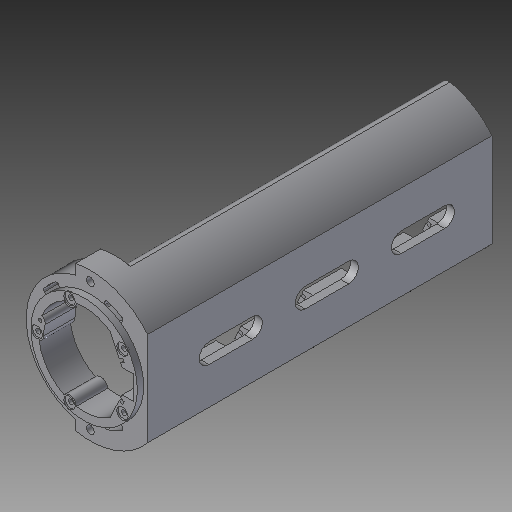
# Autodesk Inventor part: 3212_Bed Rail Base Junction_V1
Saved by Autodesk Inventor 2020 (Build 240168000, 168)
## iProperties
Created: 2019-06-18
Part Number: 3212_Bed Rail Base Junction_V1
Material: Acetal Resin, White
Document SubType Name: Sheet Metal
Designer: MPI
Density: 1.425 g/cm^3
Sheet Metal Rule: Default_mm
Appearance: Smooth - White
Mass: 1109.81 g
Surface Area: 2041.44 cm^2
Volume: 778.816 cm^3
Author: MPI
Autodesk Inventor part; units mm, degrees
ref_plane "YZ Plane" through (0, 0, 0) normal (1, 0, 0) x (0, 1, 0)
ref_plane "XZ Plane" through (0, 0, 0) normal (0, 1, 0) x (-1, 0, 0)
sketch "Sketch1" plane through (0, 0, 0) normal (0, 0, 1) x (1, 0, 0)
  circle A0 centre (0, 0) radius 54
  line L0 (48, 0) -> (-65, 0) construction
  line L1 (0, -54) -> (0, 65) construction
  dimension "d0" = 108
  constraints: 4 end point, 1 coincident, 1 horizontal, 1 perpendicular, 1 vertical alignment, 2 other
extrude "Extrusion1" add sketch "Sketch1" along normal blind 6.35
sketch "Sketch4" plane through (0, 0, 0) normal (0, 0, -1) x (-1, 0, 0)
  line L0 (15, 73.484692) -> (15, 63.245553)
  line L1 (15, -63.245553) -> (15, -73.484692)
  line L2 (-58, 47.549974) -> (-58, -47.549974)
  arc A0 (15, -63.245553) -> (15, 63.245553) centre (0, 0) ccw
  arc A1 (15, 73.484692) -> (-58, 47.549974) centre (0, 0) ccw
  arc A2 (-58, -47.549974) -> (15, -73.484692) centre (0, 0) ccw
  line L3 (-59, 0) -> (82, 0) construction
  line L4 (0, 75) -> (0, -119) construction
  line L5 (-30.377899, -43.384136) -> (-32.673725, -46.662915)
  line L6 (-13.707639, -51.157606) -> (-14.743601, -55.02387)
  line L7 (30.377899, -43.384136) -> (32.673725, -46.662915)
  line L8 (43.384136, -30.377899) -> (46.662915, -32.673725)
  line L9 (43.384136, 30.377899) -> (46.662915, 32.673725)
  line L10 (30.377899, 43.384136) -> (32.673725, 46.662915)
  line L11 (-13.707639, 51.157606) -> (-14.743601, 55.02387)
  line L12 (-30.377899, 43.384136) -> (-32.673725, 46.662915)
  arc A3 (35.51596, -47.112807) -> (47.112807, -35.51596) centre (0, 0) ccw
  arc A4 (30.808045, -40.643135) -> (40.643135, -30.808045) centre (0, 0) ccw
  arc A5 (-32.124383, -49.487615) -> (-17.260557, -56.418731) centre (0, 0) ccw
  arc A6 (-27.655082, -42.850863) -> (-15.049321, -48.729026) centre (0, 0) ccw
  arc A7 (47.112807, 35.51596) -> (35.51596, 47.112807) centre (0, 0) ccw
  arc A8 (-17.260557, 56.418731) -> (-32.124383, 49.487615) centre (0, 0) ccw
  arc A9 (40.643135, 30.808045) -> (30.808045, 40.643135) centre (0, 0) ccw
  arc A10 (-15.049321, 48.729026) -> (-27.655082, 42.850863) centre (0, 0) ccw
  arc A11 (46.662915, 32.673725) -> (47.112807, 35.51596) centre (45.515763, 34.312029) ccw
  arc A12 (40.643135, 30.808045) -> (43.384136, 30.377899) centre (42.236983, 32.016203) ccw
  arc A13 (35.51596, 47.112807) -> (32.673725, 46.662915) centre (34.312029, 45.515763) ccw
  arc A14 (30.377899, 43.384136) -> (30.808045, 40.643135) centre (32.016203, 42.236983) ccw
  arc A15 (-14.743601, 55.02387) -> (-17.260557, 56.418731) centre (-16.675453, 54.506231) ccw
  arc A16 (-15.049321, 48.729026) -> (-13.707639, 51.157606) centre (-15.639491, 50.639968) ccw
  arc A17 (-30.377899, 43.384136) -> (-27.655082, 42.850863) centre (-28.739595, 44.531289) ccw
  arc A18 (-32.124383, 49.487615) -> (-32.673725, 46.662915) centre (-31.035421, 47.810068) ccw
  arc A19 (-27.655082, -42.850863) -> (-30.377899, -43.384136) centre (-28.739595, -44.531289) ccw
  arc A20 (-32.673725, -46.662915) -> (-32.124383, -49.487615) centre (-31.035421, -47.810068) ccw
  arc A21 (-13.707639, -51.157606) -> (-15.049321, -48.729026) centre (-15.639491, -50.639968) ccw
  arc A22 (-17.260557, -56.418731) -> (-14.743601, -55.02387) centre (-16.675453, -54.506231) ccw
  arc A23 (47.112807, -35.51596) -> (46.662915, -32.673725) centre (45.515763, -34.312029) ccw
  arc A24 (43.384136, -30.377899) -> (40.643135, -30.808045) centre (42.236983, -32.016203) ccw
  arc A25 (32.673725, -46.662915) -> (35.51596, -47.112807) centre (34.312029, -45.515763) ccw
  arc A26 (30.808045, -40.643135) -> (30.377899, -43.384136) centre (32.016203, -42.236983) ccw
  circle A27 centre (0, 0) radius 48 construction
  line L13 (0, 0) -> (-41.259867, 29.977048) construction
  line L14 (0, 0) -> (-41.259867, -29.977048) construction
  arc A28 (7.840308, 45.326919) -> (20.299552, 41.278665) centre (14.832816, 45.650713) ccw
  circle A29 centre (48, 0) radius 2.5
  circle A30 centre (14.832816, 45.650713) radius 2.5
  circle A31 centre (-38.832816, 28.213692) radius 2.5
  circle A32 centre (-38.832816, -28.213692) radius 2.5
  line L15 (0, 0) -> (56.989624, 15.270324) construction
  arc A33 (41, 0) -> (39.602959, 10.611581) centre (0, 0) ccw
  arc A34 (41, 0) -> (45.53125, -6.550212) centre (48, 0) ccw
  arc A35 (20.299552, -41.278665) -> (45.53125, -6.550212) centre (0, 0) ccw
  arc A36 (45.260595, 8.214533) -> (42.72822, 17.038169) centre (0, 0) ccw construction
  arc A37 (42.877926, 16.657836) -> (20.299552, 41.278665) centre (0, 0) ccw
  circle A38 centre (44.432588, 11.905676) radius 1.75
  line L16 (-38.539425, 12) -> (-50, 12)
  line L17 (-38.539425, -12) -> (-50, -12)
  line L18 (0, 0) -> (-41.065424, 19.149122) construction
  line L19 (0, 0) -> (-39.587993, -18.460184) construction
  line L20 (0, 0) -> (7.437953, -15.950741) construction
  line L21 (0, 0) -> (6.145827, 13.179769) construction
  line L22 (-36.970763, -15.364007) -> (-40.595994, -17.05448)
  line L23 (-40.595994, -17.05448) -> (-39.159092, -20.135927)
  line L24 (-39.159092, -20.135927) -> (-35.53386, -18.445454)
  line L25 (-36.970763, 15.364007) -> (-40.595994, 17.05448)
  line L26 (-40.595994, 17.05448) -> (-39.159092, 20.135927)
  line L27 (-39.159092, 20.135927) -> (-35.53386, 18.445454)
  line L28 (-38.539425, 12) -> (-36.970763, 15.364007)
  line L29 (-35.53386, 18.445454) -> (-26.65227, 37.492086)
  line L30 (-38.539425, -12) -> (-36.970763, -15.364007)
  line L31 (-35.53386, -18.445454) -> (-26.65227, -37.492086)
  arc A39 (-26.65227, -37.492086) -> (7.840308, -45.326919) centre (0, 0) ccw
  arc A40 (7.840308, 45.326919) -> (-26.65227, 37.492086) centre (0, 0) ccw
  line L32 (-50, 12) -> (-50, -12)
  circle A41 centre (0, 65) radius 4
  circle A42 centre (0, -65) radius 4
  arc A43 (42.877926, 16.657836) -> (39.602959, 10.611581) centre (44.432588, 11.905676) ccw
  line L33 (0, 0) -> (21.950591, 67.556973) construction
  line L34 (0, 0) -> (22.421249, -69.00551) construction
  circle A44 centre (14.832816, -45.650713) radius 2.5
  arc A45 (20.299552, -41.278665) -> (7.840308, -45.326919) centre (14.832816, -45.650713) ccw
  point P0 (-33.84101, -48.329971)
  point P1 (33.84101, -48.329971)
  point P2 (48.329971, -33.84101)
  point P3 (48.329971, 33.84101)
  point P4 (33.84101, 48.329971)
  point P5 (-33.84101, 48.329971)
  point P6 (41.776754, 29.252398)
  point P7 (29.252398, 41.776754)
  point P8 (-15.270324, -56.989624)
  point P9 (29.252398, -41.776754)
  point P10 (41.776754, -29.252398)
  point P11 (-29.252398, -41.776754)
  point P12 (-29.252398, 41.776754)
  point P13 (-15.270324, 56.989624)
  point P14 (-13.199771, 49.262217)
  point P15 (-13.199771, -49.262217)
  dimension "d70" = 15
  dimension "d71" = 58
  dimension "d74" = 35
  dimension "d75" = 15
  dimension "d76" = 15
  dimension "d77" = 35
  dimension "d78" = 35
  dimension "d79" = 35
  dimension "d80" = 35
  dimension "d81" = 35
  dimension "d82" = 51
  dimension "d83" = 51
  dimension "d84" = 51
  dimension "d85" = 51
  dimension "d86" = 59
  dimension "d87" = 59
  dimension "d88" = 59
  dimension "d89" = 59
  dimension "d90" = 2
  dimension "d91" = 96
  dimension "d92" = 36
  dimension "d93" = 36
  dimension "d95" = 14
  dimension "d97" = 5
  dimension "d99" = 5
  dimension "d100" = 5
  dimension "d101" = 5
  dimension "d103" = 15
  dimension "d107" = 3.5
  dimension "d108" = 24
  dimension "d109" = 12
  dimension "d110" = 25
  dimension "d111" = 25
  dimension "d112" = 90
  dimension "d113" = 90
  dimension "d117" = 3.4
  dimension "d118" = 1.7
  dimension "d119" = 3.4
  dimension "d120" = 1.7
  dimension "d121" = 4
  dimension "d122" = 4
  dimension "d123" = 50
  dimension "d124" = 8
  dimension "d125" = 0
  dimension "d126" = 65
  dimension "d127" = 8
  dimension "d128" = 0
  dimension "d129" = 65
  dimension "d132" = 5
  dimension "d295" = 72
  dimension "d296" = 72
  dimension "d297" = 5
  dimension "d351" = 65
  dimension "d352" = 75
  dimension "d353" = 46
  dimension "d354" = 46
  dimension "d355" = 46
  dimension "d356" = 46
  dimension "d357" = 40
  dimension "d358" = 40
  constraints: 97 point on circle, 70 end point, 46 centre point, 32 tangent, 25 point on line, 15 equal radius, 11 coincident, 6 parallel, 5 perpendicular, 5 vertical, 3 horizontal, 1 collinear
  measures "d70" distance from line of point (0, 0) L0
  measures "d71" distance from line of L2 point (0, 0)
  measures "d74" angle of L5 L4
  measures "d75" angle of L6 L4
  measures "d76" angle of L4 L11
  measures "d77" angle of L4 L12
  measures "d78" angle of L9 L3
  measures "d79" angle of L4 L10
  measures "d80" angle of L4 L7
  measures "d81" angle of L8 L3
  measures "d82" radius of A9
  measures "d83" radius of A4
  measures "d84" radius of A6
  measures "d85" radius of A10
  measures "d86" radius of A8
  measures "d87" radius of A7
  measures "d88" radius of A3
  measures "d89" radius of A5
  measures "d90" radius of A11
  measures "d91" diameter of A27
  measures "d92" angle of L3 L13
  measures "d93" angle of L3 L14
  measures "d95" diameter of A28
  measures "d97" diameter of A29
  measures "d99" diameter of A30
  measures "d100" diameter of A31
  measures "d101" diameter of A32
  measures "d103" angle of L15 L3
  measures "d107" diameter of A38
  measures "d108" distance between parallel lines of L17 L16
  measures "d109" distance between parallel lines of L3 L16
  measures "d110" angle of L18 L3
  measures "d111" angle of L3 L19
  measures "d112" angle of L19 L20
  measures "d113" angle of L18 L21
  measures "d117" distance of L25.end L26.end
  measures "d118" distance between parallel lines of L18 L25
  measures "d119" distance of L22.end L23.end
  measures "d120" distance between parallel lines of L22 L19
  measures "d121" distance of L22.start L22.end
  measures "d122" distance of L25.start L25.end
  measures "d123" distance from line of L32 A0.centre
  measures "d124" diameter of A41
  measures "d125" horizontal distance of A0.centre A41.centre
  measures "d126" distance of L18.start A41.centre
  measures "d127" diameter of A42
  measures "d128" distance from line of L4 A42.centre
  measures "d129" distance of L13.start A42.centre
  measures "d132" radius of A43
  measures "d295" angle of L33 L3
  measures "d296" angle of L3 L34
  measures "d297" diameter of A44
  measures "d351" radius of A0
  measures "d352" radius of A1
  measures "d353" radius of A37
  measures "d354" radius of A40
  measures "d355" radius of A39
  measures "d356" radius of A35
  measures "d357" distance between parallel lines of L29 L21
  measures "d358" distance between parallel lines of L31 L20
extrude "Extrusion2" add sketch "Sketch4" along normal blind 25.4 contours L0 A0 L1 A2 L2 A1 | A28 A37 A43 A33 A34 A35 A45 A39 L31 L24 L23 L22 L30 L17 L32 L16 L28 L25 L26 L27 L29 A40 | A44
sketch "Sketch5" plane through (0, 0, 6.35) normal (0, 0, 1) x (1, 0, 0)
  circle A0 centre (0, 0) radius 48 construction
  line L0 (48, 0) -> (-75, 0) construction
  line L1 (0, -48) -> (0, 94) construction
  line L2 (0, 0) -> (41.489367, -30.14379) construction
  line L3 (0, 0) -> (40.486545, 29.415196) construction
  circle A1 centre (-48, 0) radius 2.5
  circle A2 centre (-48, 0) radius 2.5
  circle A3 centre (-14.832816, 45.650713) radius 2.5
  circle A4 centre (-14.832816, 45.650713) radius 2.5
  circle A5 centre (38.832816, 28.213692) radius 2.5
  circle A6 centre (38.832816, 28.213692) radius 2.5
  circle A7 centre (38.832816, -28.213692) radius 2.5
  circle A8 centre (38.832816, -28.213692) radius 2.5
  arc A9 (-45.53125, -6.550212) -> (-41, 0) centre (-48, 0) ccw
  arc A10 (-20.299552, 41.278665) -> (-7.840308, 45.326919) centre (-14.832816, 45.650713) ccw
  arc A11 (-45.53125, -6.550212) -> (-20.299552, -41.278665) centre (0, 0) ccw
  line L4 (50, -12) -> (50, 12)
  line L5 (0, 0) -> (36.093359, -16.83061) construction
  line L6 (0, 0) -> (31.707823, 14.785601) construction
  line L7 (0, 0) -> (-8.273711, -17.743031) construction
  line L8 (0, 0) -> (-8.420609, 18.058055) construction
  line L9 (35.53386, -18.445454) -> (39.159092, -20.135927)
  line L10 (39.159092, -20.135927) -> (40.595994, -17.05448)
  line L11 (40.595994, -17.05448) -> (36.970763, -15.364007)
  line L12 (35.53386, 18.445454) -> (39.159092, 20.135927)
  line L13 (39.159092, 20.135927) -> (40.595994, 17.05448)
  line L14 (40.595994, 17.05448) -> (36.970763, 15.364007)
  line L15 (26.65227, -37.492086) -> (35.53386, -18.445454)
  line L16 (36.970763, -15.364007) -> (38.539425, -12)
  line L17 (38.539425, 12) -> (36.970763, 15.364007)
  line L18 (35.53386, 18.445454) -> (26.65227, 37.492086)
  arc A12 (-7.840308, -45.326919) -> (26.65227, -37.492086) centre (0, 0) ccw
  arc A13 (26.65227, 37.492086) -> (-7.840308, 45.326919) centre (0, 0) ccw
  line L19 (50, -12) -> (50, 12)
  line L20 (0, 0) -> (-71.797599, 19.238109) construction
  arc A14 (-20.299552, 41.278665) -> (-42.877926, 16.657836) centre (0, 0) ccw
  arc A15 (-43.810195, 14.023796) -> (-44.720576, 10.773582) centre (0, 0) ccw construction
  circle A16 centre (-44.432588, 11.905676) radius 1.75
  circle A17 centre (-44.432588, 11.905676) radius 1.75
  arc A18 (-39.602959, 10.611581) -> (-42.877926, 16.657836) centre (-44.432588, 11.905676) ccw
  arc A19 (-39.602959, 10.611581) -> (-41, 0) centre (0, 0) ccw
  line L21 (0, 0) -> (-22.844489, -70.308109) construction
  circle A20 centre (-14.832816, -45.650713) radius 2.5
  arc A21 (-7.840308, -45.326919) -> (-20.299552, -41.278665) centre (-14.832816, -45.650713) ccw
  line L22 (0, 0) -> (-22.665928, 69.758553) construction
  line L23 (38.539425, -12) -> (50, -12)
  line L24 (38.539425, 12) -> (50, 12)
  point P0 (44.407207, -12)
  point P1 (44.407207, 12)
  dimension "d144" = 96
  dimension "d145" = 36
  dimension "d146" = 36
  dimension "d148" = 5
  dimension "d150" = 5
  dimension "d151" = 5
  dimension "d152" = 5
  dimension "d162" = 14
  dimension "d164" = 14
  dimension "d168" = 25
  dimension "d169" = 25
  dimension "d170" = 90
  dimension "d171" = 90
  dimension "d173" = 1.7
  dimension "d175" = 1.7
  dimension "d176" = 3.4
  dimension "d179" = 4
  dimension "d182" = 3.4
  dimension "d183" = 50
  dimension "d291" = 15
  dimension "d292" = 3.5
  dimension "d294" = 10
  dimension "d299" = 72
  dimension "d300" = 5
  dimension "d302" = 72
  dimension "d359" = 24
  dimension "d360" = 12
  dimension "d361" = 40
  dimension "d362" = 40
  dimension "d363" = 46
  dimension "d364" = 46
  dimension "d365" = 46
  dimension "d366" = 46
  dimension "d367" = 41
  constraints: 48 end point, 23 point on circle, 17 centre point, 12 coincident, 11 parallel, 3 point on line, 2 horizontal, 2 vertical, 1 equal length, 1 perpendicular
  measures "d144" diameter of A0
  measures "d145" angle of L2 L0
  measures "d146" angle of L0 L3
  measures "d148" diameter of A2
  measures "d150" diameter of A4
  measures "d151" diameter of A6
  measures "d152" diameter of A8
  measures "d162" diameter of A9
  measures "d164" diameter of A10
  measures "d168" angle of L5 L0
  measures "d169" angle of L0 L6
  measures "d170" angle of L5 L7
  measures "d171" angle of L6 L8
  measures "d173" distance between parallel lines of L5 L11
  measures "d175" distance between parallel lines of L14 L6
  measures "d176" distance of L12.end L13.end
  measures "d179" distance of L12.start L12.end
  measures "d182" distance of L9.end L10.end
  measures "d183" distance from line of L19 point (0, 0)
  measures "d291" angle of L20 L0
  measures "d292" diameter of A17
  measures "d294" diameter of A18
  measures "d299" angle of L21 L0
  measures "d300" diameter of A20
  measures "d302" angle of L22 L0
  measures "d359" distance between parallel lines of L24 L23
  measures "d360" distance between parallel lines of L0 L23
  measures "d361" distance between parallel lines of L15 L7
  measures "d362" distance between parallel lines of L18 L8
  measures "d363" radius of A11
  measures "d364" radius of A14
  measures "d365" radius of A13
  measures "d366" radius of A12
  measures "d367" radius of A19
extrude "Extrusion3" cut sketch "Sketch5" against normal up to next
sketch "Sketch6" plane through (0, 0, 6.35) normal (0, 0, 1) x (1, 0, 0)
  circle A0 centre (-48, 0) radius 5.75
  circle A1 centre (38.832816, 28.213692) radius 5.75
  circle A2 centre (38.832816, -28.213692) radius 5.75
  circle A3 centre (-48, 0) radius 2.5
  circle A4 centre (38.832816, 28.213692) radius 2.5
  circle A5 centre (38.832816, -28.213692) radius 2.5
  arc A6 (-7.840308, -45.326919) -> (-20.299552, -41.278665) centre (-14.832816, -45.650713) ccw
  circle A7 centre (-14.832816, -45.650713) radius 5.75
  circle A8 centre (-14.832816, 45.650713) radius 2.5
  circle A9 centre (-14.832816, 45.650713) radius 5.75
  point P0 (0, 0)
  dimension "d156" = 11.5
  dimension "d158" = 11.5
  dimension "d159" = 11.5
  dimension "d303" = 11.5
  dimension "d304" = 11.5
  constraints: 5 centre point, 3 concentric, 2 coincident
  measures "d156" diameter of A0
  measures "d158" diameter of A1
  measures "d159" diameter of A2
  measures "d303" diameter of A7
  measures "d304" diameter of A9
extrude "Extrusion4" cut sketch "Sketch6" against normal blind 1.5
sketch "Sketch7" plane through (0, 0, -25.4) normal (0, 0, -1) x (-1, 0, 0)
  line L0 (6.35, 68.666174) -> (6.35, 61.333826)
  line L1 (6.35, 61.333826) -> (0, 57.667652)
  line L2 (0, 57.667652) -> (-6.35, 61.333826)
  line L3 (-6.35, 61.333826) -> (-6.35, 68.666174)
  line L4 (-6.35, 68.666174) -> (0, 72.332348)
  line L5 (0, 72.332348) -> (6.35, 68.666174)
  line L6 (6.35, -61.333826) -> (6.35, -68.666174)
  line L7 (6.35, -68.666174) -> (0, -72.332348)
  line L8 (0, -72.332348) -> (-6.35, -68.666174)
  line L9 (-6.35, -68.666174) -> (-6.35, -61.333826)
  line L10 (-6.35, -61.333826) -> (0, -57.667652)
  line L11 (0, -57.667652) -> (6.35, -61.333826)
  circle A0 centre (0, -65) radius 4
  circle A1 centre (0, 65) radius 4
  point P0 (0, 0)
  dimension "d184" = 120
  dimension "d185" = 120
  dimension "d188" = 120
  dimension "d189" = 120
  dimension "d190" = 12.7
  dimension "d191" = 12.7
  constraints: 24 end point, 6 equal length, 6 parallel, 2 vertical
  measures "d184" angle of L5 L0
  measures "d185" angle of L1 L0
  measures "d188" angle of L11 L6
  measures "d189" angle of L7 L6
  measures "d190" distance between parallel lines of L9 L6
  measures "d191" distance between parallel lines of L3 L0
extrude "Extrusion5" cut sketch "Sketch7" against normal blind 5
sketch "Sketch8" plane through (0, 0, -25.4) normal (0, 0, -1) x (-1, 0, 0)
  line L0 (-14, 82) -> (-14, -73.543219) construction
  line L1 (-10.519349, 66.543219) -> (-17.480651, 66.543219) construction
  arc A0 (-20.766779, 64.751377) -> (-15.441176, 73.393256) centre (-14, 66.543219) ccw
  arc A1 (-17.480651, -65.714738) -> (-11, -67.104396) centre (0, 0) ccw construction
  arc A2 (-15.441176, -73.393256) -> (-20.766779, -64.751377) centre (-14, -66.543219) ccw
  line L2 (-58, 47.549974) -> (-58, -47.549974)
  arc A3 (-15.441176, 73.393256) -> (-58, 47.549974) centre (0, 0) ccw
  arc A4 (-58, -47.549974) -> (-15.441176, -73.393256) centre (0, 0) ccw
  arc A5 (-20.766779, 64.751377) -> (-50, 46.086874) centre (0, 0) ccw
  arc A6 (-50, -46.086874) -> (-20.766779, -64.751377) centre (0, 0) ccw
  line L3 (0, 0) -> (-83, 0) construction
  line L4 (-35.53386, 18.445454) -> (-32.011118, 26)
  line L5 (-32.011118, 26) -> (-50, 26)
  line L6 (-50, 46.086874) -> (-50, 26)
  line L7 (-35.53386, -18.445454) -> (-32.011118, -26)
  line L8 (-50, 12) -> (-50, -12)
  line L9 (-50, -26) -> (-50, -46.086874)
  line L10 (-32.011118, -26) -> (-50, -26)
  line L11 (-50, 12) -> (-38.539425, 12)
  line L12 (-40.595994, 17.05448) -> (-36.970763, 15.364007)
  line L13 (-36.970763, 15.364007) -> (-40.595994, 17.05448)
  line L14 (-40.595994, 17.05448) -> (-39.159092, 20.135927)
  line L15 (-38.539425, 12) -> (-36.970763, 15.364007)
  line L16 (-36.970763, 15.364007) -> (-38.539425, 12)
  line L17 (-39.159092, 20.135927) -> (-35.53386, 18.445454)
  line L18 (-36.970763, -15.364007) -> (-40.595994, -17.05448)
  line L19 (-35.53386, -18.445454) -> (-26.65227, -37.492086)
  line L20 (-50, 12) -> (-50, -12)
  line L21 (-50, -12) -> (-38.539425, -12)
  line L22 (-36.970763, -15.364007) -> (-38.539425, -12)
  line L23 (-35.53386, -18.445454) -> (-39.159092, -20.135927)
  line L24 (-35.53386, -18.445454) -> (-39.159092, -20.135927)
  line L25 (-36.970763, -15.364007) -> (-40.595994, -17.05448)
  line L26 (-40.595994, -17.05448) -> (-39.159092, -20.135927)
  dimension "d202" = 14
  dimension "d206" = 7
  dimension "d207" = 58
  dimension "d340" = 66.54322
  dimension "d368" = 7
  constraints: 42 end point, 15 point on circle, 7 centre point, 5 vertical, 3 horizontal, 2 coincident, 2 collinear, 2 midpoint, 2 perpendicular, 2 point on line
  measures "d202" distance from line of point (0, 0) L0
  measures "d206" radius of A2
  measures "d207" distance from line of L2 point (0, 0)
  measures "d340" distance from line of L3 A0.centre
  measures "d368" radius of A0
extrude "Extrusion6" add sketch "Sketch8" along normal blind 323.85
sketch "Sketch14" plane through (50, -12, 6.35) normal (-1, 0, 0) x (0, 0, 1)
  line L0 (-31.75, -23) -> (-57.15, -23)
  line L1 (-57.15, -23) -> (-57.15, 47)
  line L2 (-57.15, 47) -> (-31.75, 47)
  line L3 (-31.75, 47) -> (-31.75, -23)
  line L4 (-31.75, -14) -> (-355.6, -14)
  line L5 (-31.75, -25.492086) -> (-31.75, -14)
  line L6 (-95.25, 47) -> (-95.25, -23)
  line L7 (-95.25, -23) -> (-120.65, -23)
  line L8 (-120.65, -23) -> (-120.65, 47)
  line L9 (-120.65, 47) -> (-95.25, 47)
  line L10 (-158.75, 47) -> (-158.75, -23)
  line L11 (-158.75, -23) -> (-184.15, -23)
  line L12 (-184.15, -23) -> (-184.15, 47)
  line L13 (-184.15, 47) -> (-158.75, 47)
  line L14 (-222.25, 47) -> (-222.25, -23)
  line L15 (-222.25, -23) -> (-247.65, -23)
  line L16 (-247.65, -23) -> (-247.65, 47)
  line L17 (-247.65, 47) -> (-222.25, 47)
  line L18 (-285.75, 47) -> (-285.75, -23)
  line L19 (-285.75, -23) -> (-311.15, -23)
  line L20 (-311.15, -23) -> (-311.15, 47)
  line L21 (-311.15, 47) -> (-285.75, 47)
  line L22 (-349.25, 47) -> (-349.25, -23)
  line L23 (-349.25, -23) -> (-374.65, -23)
  line L24 (-374.65, -23) -> (-374.65, 47)
  line L25 (-374.65, 47) -> (-349.25, 47)
  point P0 (-6.35, 12)
  dimension "d305" = 70
  dimension "d306" = 9
  dimension "d307" = 25.4
  dimension "d310" = 63.5
  dimension "d369" = 38.1
  constraints: 48 end point, 2 collinear, 2 horizontal, 2 parallel, 1 perpendicular, 39 other
  measures "d305" distance of L0.end L1.end
  measures "d306" distance between parallel lines of L4 L0
  measures "d307" distance of L0.start L0.end
  measures "d310" distance of L2.end L6.start
  measures "d369" distance from line of L6.end L1
extrude "Extrusion11" cut sketch "Sketch14" along normal blind 38.1
sketch "Sketch15" plane through (50, -12, 6.35) normal (-1, 0, 0) x (0, 0, 1)
  line L0 (-68.75, 2) -> (-112.75, 2)
  line L1 (-112.75, 22) -> (-68.75, 22)
  line L2 (-166.175, 2) -> (-210.175, 2)
  line L3 (-210.175, 22) -> (-166.175, 22)
  line L4 (-263.6, 2) -> (-307.6, 2)
  line L5 (-307.6, 22) -> (-263.6, 22)
  line L6 (-57.15, 0) -> (-95.25, 0)
  line L7 (-31.75, 75.245553) -> (-31.75, -51.245553)
  line L8 (-355.6, -34.086874) -> (-355.6, 58.086874)
  arc A0 (-68.75, 2) -> (-68.75, 22) centre (-68.75, 12) ccw
  arc A1 (-112.75, 22) -> (-112.75, 2) centre (-112.75, 12) ccw
  arc A2 (-166.175, 2) -> (-166.175, 22) centre (-166.175, 12) ccw
  arc A3 (-210.175, 22) -> (-210.175, 2) centre (-210.175, 12) ccw
  arc A4 (-263.6, 2) -> (-263.6, 22) centre (-263.6, 12) ccw
  arc A5 (-307.6, 22) -> (-307.6, 2) centre (-307.6, 12) ccw
  point P0 (-6.35, 12)
  point P1 (-355.6, -27.086874)
  point P2 (-355.6, 51.086874)
  point P3 (-355.6, -30.836874)
  point P4 (-355.6, 54.836874)
  dimension "d320" = 20
  dimension "d321" = 2
  dimension "d324" = 44
  dimension "d327" = 37
  dimension "d328" = 48
  dimension "d370" = 53.425
  dimension "d371" = 53.425
  dimension "d372" = 44
  dimension "d373" = 44
  dimension "d374" = 44
  constraints: 12 end point, 12 point on circle, 6 centre point, 3 horizontal, 3 parallel, 3 point on line, 2 collinear, 1 tangent
  measures "d320" distance of L0.end L1.start
  measures "d321" distance between parallel lines of L0 L6
  measures "d324" distance of L0.start L0.end
  measures "d327" distance from line of L7 A0.centre
  measures "d328" distance from line of L8 A5.centre
  measures "d370" distance of A2.centre A1.centre
  measures "d371" distance of A4.centre A3.centre
  measures "d372" distance of A5.centre A4.centre
  measures "d373" distance of A3.centre A2.centre
  measures "d374" distance of A1.centre A0.centre
extrude "Extrusion13" cut sketch "Sketch15" against normal through all
ref_plane "Work Plane2" through (7, -12, 6.35) normal (-1, 0, 0) x (0, 0, 1)
sketch "Sketch16" plane through (7, -12, 6.35) normal (-1, 0, 0) x (0, 0, 1)
  line L0 (-298, 78.543) -> (-382, 78.543) construction
  line L1 (-302, -54.543) -> (-372, -54.543) construction
  line L2 (-335.2, 115) -> (-335.2, -101) construction
  line L3 (-355.6, 58.086874) -> (-355.6, 76.751377)
  arc A0 (-307.6, 22) -> (-307.6, 2) centre (-307.6, 12) ccw
  circle A1 centre (-335.2, 78.543) radius 2.5
  circle A2 centre (-335.2, -54.543) radius 2.5
  point P0 (-6.35, 12)
  point P1 (-355.6, 62.982922)
  point P2 (-355.6, 60.42326)
  dimension "d333" = 66.543
  dimension "d334" = 66.543
  dimension "d335" = 20.4
  dimension "d336" = 5
  dimension "d337" = 5
  constraints: 6 end point, 4 point on line, 2 centre point, 2 horizontal, 1 vertical
  measures "d333" distance from line of A0.centre L0
  measures "d334" distance from line of A0.centre L1
  measures "d335" distance from line of L3 L2.start
  measures "d336" diameter of A1
  measures "d337" diameter of A2
extrude "Extrusion14" cut sketch "Sketch16" against normal blind 7
sketch "Sketch17" plane through (0, 0, -349.25) normal (0, 0, -1) x (-1, 0, 0)
  arc A0 (-50, 39.086874) -> (-44.997129, 50.982922) centre (-50, 46.086874) ccw
  line L0 (-50, 46.086874) -> (-50, 35.70191)
  arc A1 (-44.997129, -50.982922) -> (-50, -39.086874) centre (-50, -46.086874) ccw
  line L1 (-50, -46.086874) -> (-50, -39.086874)
  arc A2 (-50, -46.086874) -> (-44.997129, -50.982922) centre (0, 0) ccw
  arc A3 (-44.997129, 50.982922) -> (-50, 46.086874) centre (0, 0) ccw
  dimension "d341" = 14
  dimension "d342" = 14
  dimension "d375" = 46.08687
  constraints: 8 point on circle, 4 centre point, 4 end point, 2 coincident, 1 point on line
  measures "d341" diameter of A0
  measures "d342" diameter of A1
  measures "d375" vertical distance of point (0, 0) point (-50, -46.087)
extrude "Extrusion15" add sketch "Sketch17" against normal blind 25.4
sketch "Sketch18" plane through (0, 0, -349.25) normal (0, 0, -1) x (-1, 0, 0)
  line L0 (-14, 69.043) -> (-14, 64.043)
  circle A0 centre (-14, 66.543) radius 3
  line L1 (-50, 46.086874) -> (-50, 39.086874)
  circle A1 centre (-50, 46.086874) radius 3.25
  arc A2 (-44.997129, -50.982922) -> (-50, -39.086874) centre (-50, -46.086874) ccw
  circle A3 centre (-50, -46.086874) radius 3.25
  arc A4 (-15.441176, -73.393256) -> (-20.766779, -64.751377) centre (-14, -66.543219) ccw
  circle A5 centre (-14, -66.543219) radius 3
  point P0 (0, 0)
  dimension "d345" = 6
  dimension "d346" = 6.5
  dimension "d347" = 6.5
  dimension "d348" = 6
  constraints: 4 centre point, 2 coincident, 1 midpoint
  measures "d345" diameter of A0
  measures "d346" diameter of A1
  measures "d347" diameter of A3
  measures "d348" diameter of A5
extrude "Extrusion16" cut sketch "Sketch18" against normal blind 25.4
equation "\"BendRadius\" = Thickness"
equation "\"BendReliefWidth\" = Thickness"
equation "\"BendReliefDepth\" = 0.5 * Thickness"
equation "\"CornerReliefSize\" = 4 * Thickness"
equation "\"MinimumRemnant\" = 2 * Thickness"
equation "\"TransitionRadius\" = BendRadius"
equation "\"JacobiRadiusSize\" = BendRadius"
equation "\"GapSize\" = Thickness"
equation "\"Thickness\" = 0.5"
body "Solid1"
